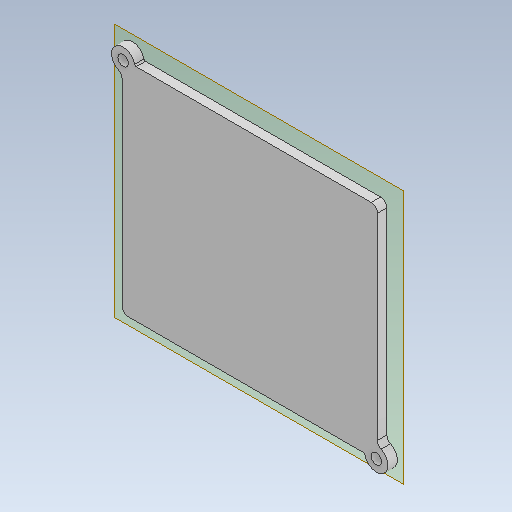
# Autodesk Inventor part: deckel
Saved by Autodesk Inventor 2021.3 (Build 253353010, 353A)
## iProperties
Created: 2021-08-02
Part Number: deckel
Material: Generisch
Document SubType Name: Modeling
Designer: Markus
Density: 1 g/cm^3
Appearance: Vorgabe
Author: Markus
Autodesk Inventor part; units mm, degrees
ref_plane "YZ Plane" through (0, 0, 0) normal (1, 0, 0) x (0, 1, 0)
ref_plane "XZ Plane" through (0, 0, 0) normal (0, 1, 0) x (-1, 0, 0)
ref_plane "XY Plane" through (0, 0, 0) normal (0, 0, 1) x (1, 0, 0)
sketch "Skizze1" plane through (0, 0, 0) normal (0, 0, 1) x (1, 0, 0)
  line L0 (-41, 29.8031) -> (-41, -33.4) projected
  arc A0 (-36.9771, 35.8002) -> (-42.1832, 31.6287) centre (-40.6517, 35.0517) ccw projected
  arc A1 (-41, 29.8031) -> (-42.1832, 31.6287) centre (-43, 29.8031) ccw projected
  line L1 (-23, 35.4) -> (-36.4872, 35.4) projected
  arc A2 (-36.9771, 35.8002) -> (-36.4872, 35.4) centre (-36.4872, 35.9) ccw projected
  line L2 (39, 35.4) -> (-8, 35.4) projected
  line L3 (41, -29.8031) -> (41, 33.4) projected
  arc A3 (41, 33.4) -> (39, 35.4) centre (39, 33.4) ccw projected
  circle A4 centre (-40.6517, 35.0517) radius 1.25 projected
  circle A5 centre (40.6517, -35.0517) radius 1.25 projected
  arc A6 (36.9771, -35.8002) -> (42.1832, -31.6287) centre (40.6517, -35.0517) ccw projected
  arc A7 (41, -29.8031) -> (42.1832, -31.6287) centre (43, -29.8031) ccw projected
  arc A8 (36.9771, -35.8002) -> (36.4872, -35.4) centre (36.4872, -35.9) ccw projected
  line L4 (35, -35.4) -> (36.4872, -35.4) projected
  arc A9 (-41, -33.4) -> (-39, -35.4) centre (-39, -33.4) ccw projected
  line L5 (-39, -35.4) -> (-35, -35.4) projected
  line L6 (-35, -35.4) -> (35, -35.4)
  line L7 (-23, 35.4) -> (-8, 35.4)
  circle A10 centre (40.6517, -35.0517) radius 1.7
  circle A11 centre (-40.6517, 35.0517) radius 1.7
  point P0 (0, 0)
  point P1 (-36.651, 36.3964)
  dimension "d6" = 3.4
  constraints: 4 end point, 2 centre point, 2 coincident, 1 collinear, 1 equal radius, 1 horizontal
  measures "d6" diameter of A10
extrude "Extrusion1" add sketch "Skizze1" along normal blind 3 contours A1 A0 A2 L1 L7 L2 A3 L3 A7 A6 A8 L4 L6 L5 A9 L0
ref_plane "Arbeitsebene1" through (0, 0, 0) normal (0, 0, -1) x (-1, 0, 0)
sketch "Skizze2" plane through (0, 0, 0) normal (0, 0, -1) x (-1, 0, 0)
  line L0 (-38, 32.1) -> (-38, -32.1) projected
  line L1 (33, -32.4) -> (-33, -32.4) projected
  line L2 (-37.7, -32.4) -> (-33, -32.4) projected
  arc A0 (-38, -32.1) -> (-37.7, -32.4) centre (-37.7, -32.1) ccw projected
  line L3 (-33, 32.4) -> (33, 32.4) projected
  line L4 (-33, 32.4) -> (-37.7, 32.4) projected
  arc A1 (-37.7, 32.4) -> (-38, 32.1) centre (-37.7, 32.1) ccw projected
  line L5 (38, -32.1) -> (38, 32.1) projected
  line L6 (33, -32.4) -> (37.7, -32.4) projected
  arc A2 (37.7, -32.4) -> (38, -32.1) centre (37.7, -32.1) ccw projected
  line L7 (37.7, 32.4) -> (33, 32.4) projected
  arc A3 (38, 32.1) -> (37.7, 32.4) centre (37.7, 32.1) ccw projected
  line L8 (-32.5, -32.2) -> (32.5, -32.2)
  line L9 (32.5, -32.2) -> (35.8, -32.2)
  line L10 (37.8, -30.2) -> (37.8, 31.2)
  line L11 (36.8, 32.2) -> (32.5, 32.2)
  line L12 (32.5, 32.2) -> (-32.5, 32.2)
  line L13 (-32.5, 32.2) -> (-36.8, 32.2)
  line L14 (-37.8, 31.2) -> (-37.8, -31.2)
  line L15 (-36.8, -32.2) -> (-32.5, -32.2)
  arc A4 (35.8, -32.2) -> (37.8, -30.2) centre (35.8, -30.2) ccw
  arc A5 (37.8, 31.2) -> (36.8, 32.2) centre (36.8, 31.2) ccw
  arc A6 (-36.8, 32.2) -> (-37.8, 31.2) centre (-36.8, 31.2) ccw
  arc A7 (-37.8, -31.2) -> (-36.8, -32.2) centre (-36.8, -31.2) ccw
  point P0 (37.8, -32.2)
  point P1 (37.8, 32.2)
  point P2 (-37.8, 32.2)
  point P3 (-37.8, -32.2)
  dimension "d7" = 0.2
  dimension "d8" = 2
  dimension "d9" = 1
  constraints: 16 end point, 8 point on circle, 8 point on line, 8 tangent, 4 centre point, 2 equal radius, 7 other
  measures "d7" distance between parallel lines of L1 L8
  measures "d8" radius of A4
  measures "d9" radius of A5
extrude "Extrusion2" add sketch "Skizze2" along normal blind 1 contours L15 A7 L14 A6 L13 L12 L11 A5 L10 A4 L9 L8
